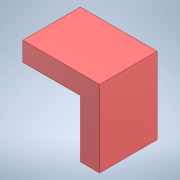
# Autodesk Inventor part: Tope_Extremos
Saved by Autodesk Inventor 2020 (Build 240168000, 168)
## iProperties
Created: 2020-07-18
Part Number: Tope_Extremos
Material: Plástico ABS
Document SubType Name: Modeling
Designer: louis
Density: 1.06 g/cm^3
Appearance: Suave - Rojo
Author: louis
Autodesk Inventor part; units mm, degrees
ref_plane "YZ Plane" through (0, 0, 0) normal (1, 0, 0) x (0, 1, 0)
ref_plane "XZ Plane" through (0, 0, 0) normal (0, 1, 0) x (-1, 0, 0)
ref_plane "XY Plane" through (0, 0, 0) normal (0, 0, 1) x (1, 0, 0)
sketch "Boceto1" plane through (0, 0, 0) normal (0, 0, 1) x (1, 0, 0)
  line L0 (-225.8925, 111.7519) -> (-185.8925, 111.7519)
  line L1 (-185.8925, 111.7519) -> (-185.8925, 71.7519)
  line L2 (-225.8925, 101.7519) -> (-195.8925, 101.7519)
  line L3 (-195.8925, 101.7519) -> (-195.8925, 71.7519)
  line L4 (-225.8925, 101.7519) -> (-225.8925, 111.7519)
  line L5 (-195.8925, 71.7519) -> (-185.8925, 71.7519)
  point P0 (0, 0)
  point P1 (0, 4.2735)
  dimension "d1" = 10
  dimension "d3" = 10
  dimension "d4" = 30
  dimension "d7" = 40
  constraints: 12 end point, 3 horizontal, 2 perpendicular
  measures "d1" distance between parallel lines of L2 L0
  measures "d3" distance between parallel lines of L1 L3
  measures "d4" distance of L2.end L3.end
  measures "d7" distance of L0.start L0.end
extrude "Extrusión1" add sketch "Boceto1" along normal blind 30
